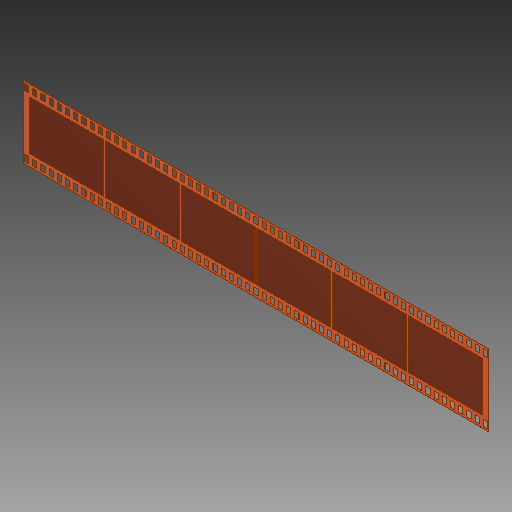
# Autodesk Inventor part: film_model_6_frames
Saved by Autodesk Inventor 2019 (Build 230136000, 136)
## iProperties
Created: 2018-10-30
Part Number: film_model_6_frames
Material: Polystyrene
Document SubType Name: Modeling
Designer: Gianpietro
Density: 1.021 g/cm^3
Appearance: Smooth - Light Orange
Mass: 0.254127 g
Surface Area: 145.697 cm^2
Volume: 0.2489 cm^3
Author: Gianpietro
Autodesk Inventor part; units mm, degrees
ref_plane "YZ Plane" through (0, 0, 0) normal (1, 0, 0) x (0, 1, 0)
ref_plane "XZ Plane" through (0, 0, 0) normal (0, 1, 0) x (-1, 0, 0)
ref_plane "XY Plane" through (0, 0, 0) normal (0, 0, 1) x (1, 0, 0)
sketch "Sketch1" plane through (0, 0, 0) normal (0, 0, 1) x (1, 0, 0)
  line L0 (-113.5, -17.5) -> (113.5, -17.5)
  line L1 (113.5, -17.5) -> (113.5, 17.5)
  line L2 (113.5, 17.5) -> (-113.5, 17.5)
  line L3 (-113.5, 17.5) -> (-113.5, -17.5)
  line L4 (-113.5, -17.5) -> (113.5, 17.5) construction
  line L5 (113.5, -17.5) -> (-113.5, 17.5) construction
  point P0 (0, 0)
  dimension "d0" = 227
  dimension "d1" = 35
  constraints: 12 end point, 2 midpoint, 2 parallel, 1 horizontal, 1 perpendicular
  measures "d0" distance of L2.end L1.end
  measures "d1" distance of L1.end L0.end
extrude "Extrusion1" add sketch "Sketch1" along normal blind 0.01
sketch "Sketch2" plane through (0, 0, 0.01) normal (0, 0, 1) x (1, 0, 0)
  line L0 (0, 0) -> (-18.5, 0)
  line L1 (-36.5, -12) -> (-0.5, -12)
  line L2 (-0.5, -12) -> (-0.5, 12)
  line L3 (-0.5, 12) -> (-36.5, 12)
  line L4 (-36.5, 12) -> (-36.5, -12)
  line L5 (-36.5, -12) -> (-0.5, 12) construction
  line L6 (-0.5, -12) -> (-36.5, 12) construction
  line L7 (-37, 0) -> (-55.5, 0)
  line L8 (-73.5, -12) -> (-37.5, -12)
  line L9 (-37.5, -12) -> (-37.5, 12)
  line L10 (-37.5, 12) -> (-73.5, 12)
  line L11 (-73.5, 12) -> (-73.5, -12)
  line L12 (-73.5, -12) -> (-37.5, 12) construction
  line L13 (-37.5, -12) -> (-73.5, 12) construction
  line L14 (-74, 0) -> (-92.5, 0)
  line L15 (-110.5, -12) -> (-74.5, -12)
  line L16 (-74.5, -12) -> (-74.5, 12)
  line L17 (-74.5, 12) -> (-110.5, 12)
  line L18 (-110.5, 12) -> (-110.5, -12)
  line L19 (-110.5, -12) -> (-74.5, 12) construction
  line L20 (-74.5, -12) -> (-110.5, 12) construction
  line L21 (74, 0) -> (55.5, 0)
  line L22 (37.5, -12) -> (73.5, -12)
  line L23 (73.5, 12) -> (37.5, 12)
  line L24 (37.5, 12) -> (37.5, -12)
  line L25 (37.5, -12) -> (73.5, 12) construction
  line L26 (73.5, -12) -> (37.5, 12) construction
  line L27 (36.5, -12) -> (36.5, 12)
  line L28 (37, 0) -> (18.5, 0)
  line L29 (36.5, 12) -> (0.5, 12)
  line L30 (0.5, -12) -> (36.5, -12)
  line L31 (0.5, 12) -> (0.5, -12)
  line L32 (0.5, -12) -> (36.5, 12) construction
  line L33 (36.5, -12) -> (0.5, 12) construction
  line L34 (73.5, -12) -> (73.5, 12)
  line L35 (111, 0) -> (92.5, 0)
  line L36 (74.5, 12) -> (74.5, -12)
  line L37 (74.5, -12) -> (110.5, -12)
  line L38 (110.5, -12) -> (110.5, 12)
  line L39 (74.5, -12) -> (110.5, 12) construction
  line L40 (110.5, -12) -> (74.5, 12) construction
  line L41 (110.5, 12) -> (74.5, 12)
  dimension "d4" = 18.5
  dimension "d5" = 36
  dimension "d6" = 24
  dimension "d9" = 37
  dimension "d16" = 111
  constraints: 84 end point, 12 midpoint, 4 horizontal, 2 collinear, 2 parallel, 1 perpendicular, 63 other
  measures "d4" distance of L0.start L0.end
  measures "d5" distance of L3.end L2.end
  measures "d6" distance of L2.end L1.end
  measures "d9" distance of L0.end L7.end
  measures "d16" distance of L7.start L21.start
extrude "Extrusion2" add sketch "Sketch2" along normal blind 0.01
mirror "Mirror1" about plane through (0, 0, 0) normal (0, 0, 1) of "Extrusion2"
mirror "Mirror2" about plane through (0, 0, 0) normal (0, 0, 1) of "Extrusion1"
sketch "Sketch3" plane through (0, 0, 0.01) normal (0, 0, 1) x (1, 0, 0)
  line L0 (0, 0) -> (0, 15)
  line L1 (-1, 13.5) -> (1, 13.5)
  line L2 (1, 13.5) -> (1, 16.5)
  line L3 (1, 16.5) -> (-1, 16.5)
  line L4 (-1, 16.5) -> (-1, 13.5)
  line L5 (-1, 13.5) -> (1, 16.5) construction
  line L6 (1, 13.5) -> (-1, 16.5) construction
  dimension "d23" = 15
  dimension "d24" = 2
  dimension "d25" = 3
  constraints: 14 end point, 2 midpoint, 2 parallel, 1 horizontal, 1 perpendicular, 1 vertical
  measures "d23" distance of L0.start L0.end
  measures "d24" distance of L3.end L2.end
  measures "d25" distance of L2.end L1.end
extrude "Extrusion3" cut sketch "Sketch3" against normal blind 0.02
pattern_linear "Rectangular Pattern1" count 57 spacing 4 along (-1, 0, 0) of "Extrusion3"
mirror "Mirror3" about plane through (0, 0, 0) normal (0, 1, 0) of "Extrusion3", "Rectangular Pattern1"
body "Solid1"
